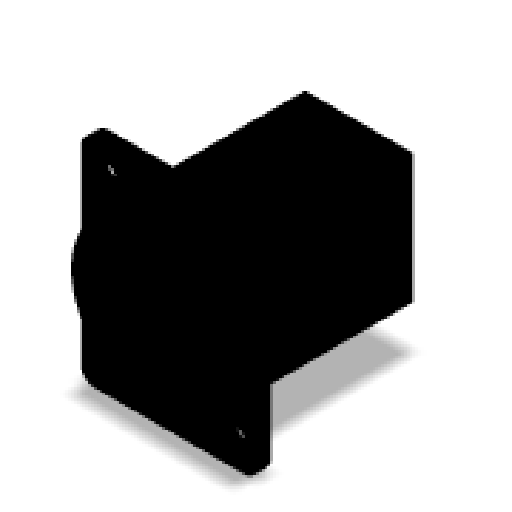
# Autodesk Inventor part: Delock Panel Connector
Saved by Autodesk Inventor 2023.2 (Build 272271000, 271)
## iProperties
Created: 2023-02-25
Part Number: Delock Panel Connector
Material: Aluminum 6061
Document SubType Name: Modeling
Designer: remop
Density: 2.7 g/cm^3
Appearance: Anodized - Black
Author: remop
Autodesk Inventor part; units mm, degrees
ref_plane "YZ Plane" through (0, 0, 0) normal (1, 0, 0) x (0, 1, 0)
ref_plane "XZ Plane" through (0, 0, 0) normal (0, 1, 0) x (-1, 0, 0)
ref_plane "XY Plane" through (0, 0, 0) normal (0, 0, 1) x (1, 0, 0)
sketch "Sketch1" plane through (0, 0, 0) normal (0, 0, 1) x (1, 0, 0)
  line L0 (13, -16) -> (-13, -16)
  line L1 (-13, -16) -> (-13, 16)
  line L2 (-13, 16) -> (13, 16)
  line L3 (13, 16) -> (13, -16)
  line L4 (13, -16) -> (-13, 16) construction
  line L5 (-13, -16) -> (13, 16) construction
  circle A0 centre (-9.5, 12) radius 1.6
  circle A1 centre (9.5, -12) radius 1.6
  point P0 (0, 0)
  dimension "d0" = 32
  dimension "d1" = 26
  dimension "d3" = 12
  dimension "d4" = 12
  dimension "d5" = 9.5
  dimension "d6" = 9.5
  dimension "d7" = 3.2
  constraints: 12 end point, 2 centre point, 2 midpoint, 2 parallel, 1 equal radius, 1 horizontal, 1 perpendicular
  measures "d0" distance of L0.end L1.end
  measures "d1" distance of L1.end L2.end
  measures "d3" vertical distance of point (0, 0) A0.centre
  measures "d4" vertical distance of point (0, 0) A1.centre
  measures "d5" horizontal distance of point (0, 0) A0.centre
  measures "d6" horizontal distance of point (0, 0) A1.centre
  measures "d7" diameter of A0
extrude "Extrusion1" add sketch "Sketch1" along normal blind 2
sketch "Sketch2" plane through (0, 0, 2) normal (0, 0, 1) x (1, 0, 0)
  circle A0 centre (0, 0) radius 12
  dimension "d10" = 24
  constraints: 1 centre point, 1 coincident
  measures "d10" diameter of A0
extrude "Extrusion2" add sketch "Sketch2" along normal blind 2.5
fillet "Fillet1" radius 2 4 edges at (-13, 16, 1) (13, 16, 1) (-13, -16, 1) (13, -16, 1)
sketch "Sketch3" plane through (0, 0, 0) normal (0, 0, -1) x (-1, 0, 0)
  line L0 (8, -9.5) -> (-8, -9.5)
  line L1 (-8, -9.5) -> (-8, 9.5)
  line L2 (-8, 9.5) -> (8, 9.5)
  line L3 (8, 9.5) -> (8, -9.5)
  line L4 (8, -9.5) -> (-8, 9.5) construction
  line L5 (-8, -9.5) -> (8, 9.5) construction
  point P0 (0, 0)
  dimension "d14" = 19
  dimension "d15" = 16
  constraints: 12 end point, 2 midpoint, 2 parallel, 1 horizontal, 1 perpendicular
  measures "d14" distance of L0.end L1.end
  measures "d15" distance of L0.start L0.end
extrude "Extrusion3" add sketch "Sketch3" along normal blind 26
sketch "Sketch4" plane through (0, 0, 4.5) normal (0, 0, 1) x (1, 0, 0)
  line L0 (6.5, -2.5) -> (-6.5, -2.5)
  line L1 (-6.5, -2.5) -> (-6.5, 2.5)
  line L2 (-6.5, 2.5) -> (6.5, 2.5)
  line L3 (6.5, 2.5) -> (6.5, -2.5)
  line L4 (6.5, -2.5) -> (-6.5, 2.5) construction
  line L5 (-6.5, -2.5) -> (6.5, 2.5) construction
  point P0 (0, 0)
  dimension "d18" = 13
  dimension "d19" = 5
  constraints: 12 end point, 2 midpoint, 2 parallel, 1 horizontal, 1 perpendicular
  measures "d18" distance of L1.end L2.end
  measures "d19" distance of L0.end L1.end
extrude "Extrusion4" cut sketch "Sketch4" against normal blind 10
equation "\"d4\" = d3"
equation "\"d6\" = d5"
body "Solid1"
